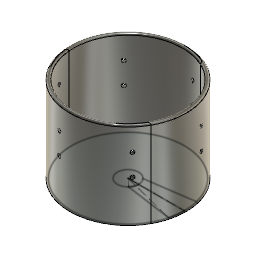
modified_drum (6) (Autodesk Fusion 360 design; units mm, degrees)
Autodesk Fusion 360 part; units mm, degrees
sketch "Sketch1" plane through (0, 0, 0) normal (0, 0, 1) x (1, 0, 0)
  arc A0 (96.5614, 31.5984) -> (-2.3405, 101.573) centre (0, 0) ccw
  line L0 (0, 0) -> (96.5614, 31.5984) construction
  line L1 (0, 0) -> (-2.3405, 101.573) construction
  arc A1 (93.7102, 30.6654) -> (-2.2714, 98.5738) centre (0, 0) ccw
  arc A2 (90.8589, 29.7324) -> (-2.2023, 95.5746) centre (0, 0) ccw
  line L2 (-2.3405, 101.573) -> (-2.2023, 95.5746)
  line L3 (96.5614, 31.5984) -> (90.8589, 29.7324)
  arc A3 (43.0665, 92.0208) -> (-2.3405, 101.573) centre (0, 0) ccw
  line L4 (0, 0) -> (43.0665, 92.0208) construction
  line L5 (0, 0) -> (-2.3405, 101.573) construction
  line L6 (43.0665, 92.0208) -> (40.5232, 86.5865)
  line L7 (-2.3405, 101.573) -> (0.776, 98.5969)
  line L8 (-2.3405, 101.573) -> (-129.4268, 101.573) construction
  line L9 (40.5232, 86.5865) -> (39.0991, 90.5164)
  arc A4 (58.1591, -83.3071) -> (96.5614, 31.5984) centre (0, 0) ccw
  arc A5 (54.7245, -78.3874) -> (90.8589, 29.7324) centre (0, 0) ccw
  line L10 (0, 0) -> (58.1591, -83.3071) construction
  line L11 (0, 0) -> (58.1591, -83.3071) construction
  line L12 (0, 0) -> (89.1351, -48.7596) construction
  line L13 (58.1591, -83.3071) -> (58.9133, -79.0644)
  arc A6 (56.4418, -80.8473) -> (93.7102, 30.6654) centre (0, 0) ccw
  line L14 (58.1591, -83.3071) -> (54.7245, -78.3874)
  line L15 (0, 0) -> (96.5614, 31.5984) construction
  line L16 (83.8712, -45.8801) -> (85.0458, -49.8916)
  line L17 (58.1591, -83.3071) -> (-44.342, -158.4366) construction
  line L18 (89.1351, -48.7596) -> (83.8712, -45.8801)
  line L19 (96.5614, 31.5984) -> (90.8589, 29.7324)
  arc A7 (58.1591, -83.3071) -> (89.1351, -48.7596) centre (0, 0) ccw
  line L20 (89.1351, -48.7596) -> (84.9995, -49.9705)
  line L21 (54.7245, -78.3874) -> (58.84, -79.119)
  dimension "d1" = 101.6
  dimension "d2" = 73.2
  dimension "d5" = 26.4
  dimension "d7" = 45
  dimension "d8" = 45
  dimension "d9" = 45
  dimension "d12" = 45
  constraint coincident A0.centre L0.start
  constraint parallel L1 L2
  constraint parallel L0 L3
  constraint coincident A1.start L3
  constraint coincident A1.end L2
  constraint coincident L4 L6.end
  constraint coincident A2 L6.end
  constraint horizontal L8
  constraint coincident A1 L7.end
  constraint coincident A1 L9.end
  constraint symmetric A0.centre L3 L0.start
  constraint symmetric A0.start L3 L0.end
  constraint symmetric A0.end L3 A4.start
  constraint symmetric A0 L3 A4
  constraint symmetric A1.start L3 A6.end
  constraint symmetric A1.end L3 A6.start
  constraint symmetric A1 L3 A6
  constraint symmetric A2.start L3 A5.end
  constraint symmetric A2.end L3 A5.start
  constraint symmetric A2 L3 A5
  constraint symmetric L3 A3.start L12.end
  constraint symmetric L3 A3 A7
  constraint symmetric L3 L6.end L16.start
  constraint symmetric L3 L7.end L13.end
  constraint symmetric L3 L8.end L17.end
  constraint symmetric L3 L9.end L16.end
  constraint coincident A6 L20.end
  constraint coincident A6 L21.end
  measures "d1" radius of A0
  measures "d2" angle of L0 L1
  measures "d5" angle of L4 L5
  measures "d7" angle of L6 L9
  measures "d8" angle of L18 L20
  measures "d9" angle of L14 L21
  measures "d12" angle of L2 L7
extrude "Extrude1" add sketch "Sketch1" along normal blind 152.4 contours A0 A1 L3 L6 L19 | L3 A4 A6 L18 L19 | A0 A1 A3 L6 L7 | A1 A2 L3 L6 L19 | L3 A5 A6 L18 L19 | A6 L18 L20 | A1 L6 L9 | A6 L16 L18 | A5 A6 L16 L21 makes body 1
fillet "Fillet1" radius 3 2 edges at (95.2478, 8.1991, 152.4) (86.7946, 52.8134, 152.4) on bodies 1
ref_plane "WorkPlane1" through (96.5614, 31.5984, 0) normal (0.950407, 0.311008, 0) x (-0.311008, 0.950407, 0)
sketch "Sketch2" plane through (96.5614, 31.5984, 0) normal (0.950407, 0.311008, 0) x (-0.311008, 0.950407, 0)
  line L0 (0, 149.4) -> (0, 111.3)
  line L1 (0, 111.3) -> (0, 73.2)
  line L2 (97.2637, 149.4) -> (-74.0632, 149.4)
  dimension "d24" = 38.1
  dimension "d25" = 38.1
  constraint vertical L0
  constraint parallel L0 L1
  constraint coincident L0.start L2
  measures "d24" distance of L0.start L0.end
  measures "d25" distance of L0.end L1.end
hole "Hole1" at (96.5614, 31.5984, 111.3) at (96.5614, 31.5984, 73.2) direction (-0.950407, -0.311008, 0) diameter 6.35 depth 12.7 tip angle 118 bodies 1
pattern_circular "C-Pattern2" count 6 over 360 about axis through (0, 0, 149.4) along (0, 0, 1) of "Hole1"
pattern_circular "C-Pattern3" count 3 over 360 about axis through (0, 0, 149.4) along (0, 0, 1) of bodies 1 makes body 2 at (-90.1076, -46.9381, 74.2725) makes body 3 at (85.7033, -54.5665, 74.2737)
sketch "Sketch1 (2)" plane through (0, 0, 0) normal (0, 0, 1) x (1, 0, 0) in component "Component"
  circle A0 centre (0, 0) radius 98.6
  circle A1 centre (0, 0) radius 18.5
  line L0 (0, 0) -> (98.6, 0)
  arc A2 (95.5348, -24.394) -> (98.6, 0) centre (0, 0) ccw
  line L1 (0, 0) -> (95.5348, -24.394) construction
  line L2 (0, 0) -> (98.6, 0) construction
  arc A3 (13.5362, -12.6103) -> (18.5, 0) centre (0, 0) ccw
  line L3 (0, 0) -> (13.5362, -12.6103) construction
  line L4 (0, 0) -> (18.5, 0) construction
  line L5 (95.5348, -24.394) -> (13.5362, -12.6103)
  line L6 (95.5348, 24.394) -> (13.5362, 12.6103)
  dimension "d38" = 197.2
  dimension "d39" = 37
  dimension "d40" = 14.324
  dimension "d41" = 42.972
  constraint coincident A0.centre A1.centre
  constraint coincident A0 L0.end
  constraint horizontal L0
  constraint coincident A1 A3.end
  constraint coincident L2 A3.end
  constraint symmetric A2.start L2 L6.start
  constraint symmetric L2 A3.start L6.end
  measures "d38" diameter of A0
  measures "d39" diameter of A1
  measures "d40" angle of L1 L2
  measures "d41" angle of L3 L4
extrude "Extrude1'" add sketch "Sketch1 (2)" along normal blind 5.08 separate body contours A0 A1 L0 L6 | A0 A1 L0 A2 A3 L5 | A1 A3 makes body 4 in component "Component"
sketch "Sketch3" plane through (0, 0, 5.08) normal (0, 0, 1) x (-1, 0, 0)
  arc A0 (-95.5348, 24.394) -> (-95.5348, -24.394) centre (0, 0) ccw
  line L0 (-95.5348, -24.394) -> (-13.5362, -12.6103)
  arc A1 (-13.5362, -12.6103) -> (-13.5362, 12.6103) centre (0, 0) ccw
  line L1 (-13.5362, 12.6103) -> (-95.5348, 24.394)
  circle A2 centre (0, 0) radius 18.5
  circle A3 centre (0, 0) radius 98.6
  circle A4 centre (0, 0) radius 93.52
  dimension "d44" = -5.08
extrude "Extrude2" add sketch "Sketch3" along normal blind 50.8 contours A0 L0 L1 A3 A4 bodies 4 in component "Component"
fillet "Fillet1'" offset 51.6 second offset 50.8 1 edges at (93.52, 0, 5.08) measured on face at (40.1975, 0, 5.08) on bodies 4 in component "Component"
shell "Shell1" thickness 2.54 removed faces 2 at (1.5737, -0.9183, 5.08) at (73.2296, 13.5731, 16.468) on bodies 4 in component "Component"
sketch "Sketch4" plane through (0, 0, 2.54) normal (0, 0, 1) x (-1, 0, 0)
  arc A0 (-93.6112, 21.5515) -> (-93.6112, -21.5515) centre (0, 0) ccw
  line L0 (-93.6112, -21.5515) -> (-12.5199, -9.8982)
  arc A1 (-12.5199, -9.8982) -> (-12.5199, 9.8982) centre (0, 0) ccw
  line L1 (-12.5199, 9.8982) -> (-93.6112, 21.5515)
  circle A2 centre (0, 0) radius 18.5
  circle A3 centre (0, 0) radius 15.96
  dimension "d51" = -2.54
extrude "Extrude3" add sketch "Sketch4" along normal blind 6.35 contours A1 A3 bodies 4 in component "Component"
fillet "Fillet2" radius 3.81 1 edges at (-15.96, 0, 5.08) on bodies 4 in component "Component"
ref_plane "WorkPlane2" through (98.6, 0, 27.94) normal (1, 0, 0) x (0, 1, 0)
sketch "Sketch5" plane through (98.6, 0, 0) normal (1, 0, 0) x (0, 1, 0)
  line L0 (0, 55.88) -> (0, 49.53)
  line L1 (0, 49.53) -> (0, 11.43)
  line L2 (0, 11.43) -> (0, 5.08)
  circle A0 centre (0, 8.255) radius 3.175
  circle A1 centre (0, 46.355) radius 3.175
  line L3 (0, 8.255) -> (-3.175, 8.255)
  line L4 (0, 8.255) -> (3.175, 8.255)
  line L5 (0, 46.355) -> (3.175, 46.355)
  line L6 (0, 46.355) -> (-3.175, 46.355)
  line L7 (3.175, 46.355) -> (3.175, 8.255)
  line L8 (-3.175, 8.255) -> (-3.175, 46.355)
  dimension "d57" = 6.35
  dimension "d58" = 38.1
  dimension "d59" = 6.35
  dimension "d60" = 6.35
  constraint vertical L0
  constraint parallel L0 L1
  constraint parallel L1 L2
  constraint coincident L2.end A0
  constraint coincident L1.end A0
  constraint coincident L0.end A1
  constraint coincident A0.centre L3.start
  constraint coincident A0 L3.end
  constraint perpendicular L2 L3
  constraint coincident A0 L4.end
  constraint perpendicular L2 L4
  constraint coincident A1.centre L5.start
  constraint coincident A1 L5.end
  constraint perpendicular L1 L5
  constraint coincident A1 L6.end
  constraint perpendicular L1 L6
  constraint tangent A0 L7
  constraint tangent A1 L8
  measures "d57" distance of L0.start L0.end
  measures "d58" distance of L0.end L1.end
  measures "d59" distance of L1.end L2.end
  measures "d60" diameter of A1
extrude "Extrude4" cut sketch "Sketch5" against normal blind 5.08 bodies 4 in component "Component"
component "Component" placed x (1, 0, 0) y (0, 1, 0) z (0, 0, 1) at (0, 0, 0)
equation "d1 = ShellDiam / 2"
equation "d2 = PieceSize * LapSize + PieceSize"
equation "d3 = -HalfShellThick"
equation "d4 = -ShellThick"
equation "d5 = PieceSize * ( LapSize * 2 )"
equation "d10 = ShellHeight"
equation "NumSegments = 3"
equation "ShellThick = 6 mm"
equation "ShellHeight = 6 in"
equation "ShellDiam = 8 in"
equation "LapSize = LapSizePercent / 100"
equation "PieceSize = ( 180 / NumSegments ) * 1 deg"
equation "d22 = HalfShellThick"
equation "d24 = LugTopDist"
equation "d25 = LugSpacing"
equation "d27 = LugHoleDiam"
equation "d29 = NumSegments * 2"
equation "d31 = NumSegments"
equation "LugTopDist = 1.5 in"
equation "LugSpacing = 1.5 in"
equation "LapSizePercent = 22"
equation "HalfShellThick = ShellThick / 2"
equation "LugHoleDiam = 0.25 in"
equation "d38 = ShellDiam - ShellThick"
equation "d40 = ( ( 360 * 1 in ) / ( PI * ShellDiam ) ) * 1 deg"
equation "d41 = ( ( 360 * 3 in ) / ( PI * ShellDiam ) ) * 1 deg"
equation "d45 = LugSpacing + ( LugHoleDiam * 2 )"
equation "d48 = ShellDiam / 2 - 50 mm"
equation "d49 = LugSpacing + ( LugHoleDiam * 2 )"
equation "d57 = LugHoleDiam"
equation "d58 = LugSpacing"
equation "d59 = LugHoleDiam"
equation "d60 = LugHoleDiam"
